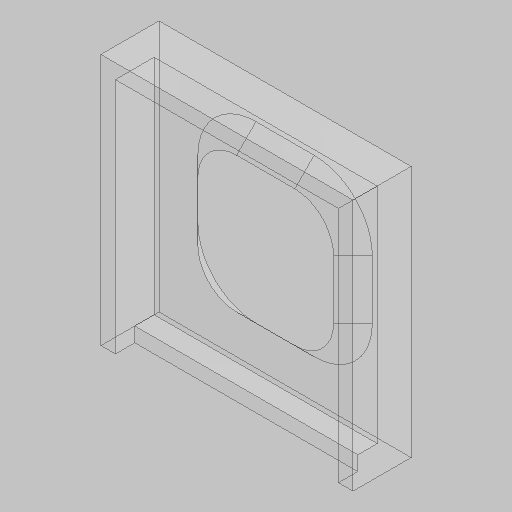
# Autodesk Inventor part: Optical module_lid
Saved by Autodesk Inventor 2026.1 (Build 301233020, 233B)
## iProperties
Created: 2026-01-23
Part Number: Optical module_lid
Material: PET Plastic
Document SubType Name: Modeling
Designer: samuel
Density: 1.541 g/cm^3
Appearance: Polycarbonate - Clear
Author: samuel
Autodesk Inventor part; units mm, degrees
ref_plane "YZ Plane" through (0, 0, 0) normal (1, 0, 0) x (0, 1, 0)
ref_plane "XZ Plane" through (0, 0, 0) normal (0, 1, 0) x (-1, 0, 0)
ref_plane "XY Plane" through (0, 0, 0) normal (0, 0, 1) x (1, 0, 0)
sketch "Sketch2" plane through (0, 0, 0) normal (0, 0, 1) x (1, 0, 0)
  line L0 (-6.5, -6.5) -> (6.5, -6.5)
  line L1 (6.5, -6.5) -> (6.5, 6.5)
  line L2 (6.5, 6.5) -> (-6.5, 6.5)
  line L3 (-6.5, 6.5) -> (-6.5, -6.5)
  line L4 (-6.5, -6.5) -> (6.5, 6.5) construction
  line L5 (6.5, -6.5) -> (-6.5, 6.5) construction
  line L6 (-5.25, -5.25) -> (5.25, -5.25)
  line L7 (5.25, -5.25) -> (5.25, 5.25)
  line L8 (5.25, 5.25) -> (-5.25, 5.25)
  line L9 (-5.25, 5.25) -> (-5.25, -5.25)
  line L10 (-5.25, -5.25) -> (5.25, 5.25) construction
  line L11 (5.25, -5.25) -> (-5.25, 5.25) construction
  line L12 (-5.75, 5.75) -> (5.75, 5.75)
  line L13 (5.75, 5.75) -> (5.75, -5.75)
  line L14 (5.75, -5.75) -> (-5.75, -5.75)
  line L15 (-5.75, -5.75) -> (-5.75, 5.75)
  line L16 (-3.5, -3.5) -> (3.5, -3.5)
  line L17 (3.5, -3.5) -> (3.5, 3.5)
  line L18 (3.5, 3.5) -> (-3.5, 3.5)
  line L19 (-3.5, 3.5) -> (-3.5, -3.5)
  line L20 (-3.5, -3.5) -> (3.5, 3.5) construction
  line L21 (3.5, -3.5) -> (-3.5, 3.5) construction
  point P0 (0, 0)
  dimension "d0" = 13
  dimension "d1" = 13
  dimension "d2" = 10.5
  dimension "d3" = 10.5
  dimension "d4" = 0.5
  dimension "d5" = 7
  dimension "d6" = 7
  constraints: 44 end point, 8 parallel, 6 midpoint, 4 perpendicular, 3 horizontal, 3 other
  measures "d0" distance of L2.end L1.end
  measures "d1" distance of L1.end L0.end
  measures "d2" distance of L8.end L7.end
  measures "d3" distance of L7.end L6.end
  measures "d4" distance between parallel lines of L8 L12
  measures "d5" distance of L18.end L17.end
  measures "d6" distance of L17.end L16.end
extrude "Extrusion1" add sketch "Sketch2" along normal blind 3 contours L3 L2 L1 L0
extrude "Extrusion2" add sketch "Sketch2" along normal blind 1 contours L9 L8 L7 L6 | L12 L13 L14 L15 | L19 L18 L17 L16
extrude "Extrusion3" cut sketch "Sketch2" along normal blind 1 contours L19 L18 L17 L16
fillet "Fillet1" radius 2 4 edges at (-3.5, 3.5, 0.5) (-3.5, -3.5, 0.5) (3.5, 3.5, 0.5) (3.5, -3.5, 0.5)
chamfer "Chamfer1" distance 1 angle 45 8 edges at (0, 3.5, 0) (-2.9142, 2.9142, 0) (-3.5, 0, 0) (-2.9142, -2.9142, 0) (0, -3.5, 0) (2.9142, -2.9142, 0) (3.5, 0, 0) (2.9142, 2.9142, 0)
sketch "Sketch3" plane through (0, 0, 3) normal (0, 0, 1) x (1, 0, 0)
  line L0 (5.75, -5.75) -> (-5.75, -5.75) projected
  line L1 (-6.5, -6.5) -> (6.5, -6.5) projected
  line L2 (-5.75, -5.75) -> (5.75, -5.75)
  line L3 (5.75, -5.75) -> (5.75, -6.5)
  line L4 (5.75, -6.5) -> (-5.75, -6.5)
  line L5 (-5.75, -6.5) -> (-5.75, -5.75)
  point P0 (0, 0)
  dimension "d17" = 11.5
  constraints: 8 end point, 2 parallel, 1 horizontal, 1 perpendicular, 1 point on line
  measures "d17" distance of L3.end L4.end
extrude "Extrusion4" cut sketch "Sketch3" against normal blind 1
body "Solid1"
